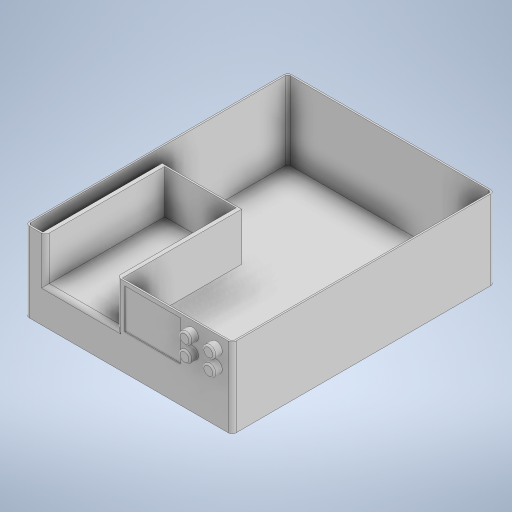
# Autodesk Inventor part: case_botten
Saved by Autodesk Inventor 2023 (Build 270158000, 158)
## iProperties
Created: 2022-12-13
Part Number: case_botten
Material: Generic
Document SubType Name: Modeling
Designer: abdul
Density: 1 g/cm^3
Appearance: Default
Author: abdul
Autodesk Inventor part; units mm, degrees
ref_plane "YZ Plane" through (0, 0, 0) normal (1, 0, 0) x (0, 1, 0)
ref_plane "XZ Plane" through (0, 0, 0) normal (0, 1, 0) x (-1, 0, 0)
ref_plane "XY Plane" through (0, 0, 0) normal (0, 0, 1) x (1, 0, 0)
sketch "Sketch1" plane through (0, 0, 0) normal (0, 1, 0) x (-1, 0, 0)
  line L0 (130, 165) -> (-130, 165)
  line L1 (-130, 165) -> (-130, -165)
  line L2 (-130, -165) -> (130, -165)
  line L3 (130, -165) -> (130, 165)
  point P0 (0, 0)
  point P1 (0, -165)
  point P2 (130, 0)
  dimension "d0" = 260
  dimension "d1" = 330
  constraints: 8 end point, 2 midpoint, 2 parallel, 1 horizontal, 1 horizontal alignment, 1 perpendicular, 1 vertical alignment
  measures "d0" distance of L2.end L1.end
  measures "d1" distance of L1.end L0.end
extrude "Extrusion1" add sketch "Sketch1" along normal blind 100
fillet "Fillet1" radius 5 4 edges at (130, 50, 165) (130, 50, -165) (-130, 50, -165) (-130, 50, 165)
shell "Shell1" thickness 2 removed faces 1 at (43.3333, 100, 53.3333)
sketch "Sketch3" plane through (128, 96, 163) normal (0, 0, -1) x (-1, 0, 0)
  line L0 (251.5, 4) -> (4.5, 4) projected
  line L1 (138, 4) -> (238, 4)
  line L2 (238, 4) -> (238, -56)
  line L3 (238, -56) -> (138, -56)
  line L4 (138, -56) -> (138, 4)
  line L5 (253, -96) -> (253, 4) projected
  point P0 (128, -96)
  point P1 (253, 2)
  dimension "d13" = 100
  dimension "d14" = 60
  dimension "d15" = 15
  constraints: 8 end point, 2 parallel, 1 horizontal, 1 perpendicular, 1 point on line
  measures "d13" distance of L2.end L3.end
  measures "d14" distance of L1.end L2.end
  measures "d15" distance between parallel lines of L2 L5
extrude "Extrusion3" add sketch "Sketch3" along normal blind 150
sketch "Sketch4" plane through (-125, 0, 165) normal (0, 0, 1) x (1, 0, 0)
  line L0 (0, 0) -> (0, 100) projected
  line L1 (0, 0) -> (250, 0) projected
  line L2 (250, 100) -> (250, 0) projected
  line L3 (15, 100) -> (115, 100) projected
  line L4 (15, 40) -> (15, 100) projected
  line L5 (15, 100) -> (115, 100) projected
  line L6 (115, 100) -> (115, 40) projected
  line L7 (115, 40) -> (15, 40) projected
  line L8 (20, 45) -> (110, 45)
  line L9 (110, 45) -> (110, 109.7523)
  line L10 (110, 109.7523) -> (20, 109.7523)
  line L11 (20, 109.7523) -> (20, 45)
  line L12 (0, 100) -> (250, 100) projected
  line L13 (0, 100) -> (-3, 100) projected
  line L14 (-3, 100) -> (0, 100) projected
  line L15 (0, 100) -> (250, 100) projected
  line L16 (250, 100) -> (253, 100) projected
  line L17 (253, 100) -> (250, 100) projected
  line L18 (250, 100) -> (115, 100) projected
  line L19 (15, 100) -> (0, 100) projected
  point P0 (125, 0)
  dimension "d18" = 5
  dimension "d19" = 5
  dimension "d20" = 5
  constraints: 8 end point, 2 parallel, 1 horizontal, 1 perpendicular
  measures "d18" distance between parallel lines of L8 L7
  measures "d19" distance between parallel lines of L4 L11
  measures "d20" distance between parallel lines of L6 L9
extrude "Extrusion4" cut sketch "Sketch4" against normal blind 150 contours L11 L10 L9 L3 | L3 L9 L8 L11
fillet "Fillet3" radius 5 3 edges at (-60, 45, 165) (-105, 72.5, 165) (-15, 72.5, 165)
sketch "Sketch5" plane through (-125, 0, 165) normal (0, 0, 1) x (1, 0, 0)
  circle A0 centre (235, 85) radius 7.5
  line L0 (115, 100) -> (250, 100) projected
  line L1 (250, 100) -> (250, 0) projected
  circle A1 centre (205, 85) radius 7.5
  circle A2 centre (235, 65) radius 7.5
  circle A3 centre (205, 65) radius 7.5
  point P0 (125, 0)
  dimension "d24" = 15
  dimension "d25" = 15
  dimension "d26" = 15
  dimension "d29" = 30
  dimension "d32" = 20
  constraints: 4 centre point, 1 horizontal, 1 vertical, 6 other
  measures "d24" diameter of A0
  measures "d25" distance from line of L0 A0.centre
  measures "d26" distance from line of L1 A0.centre
  measures "d29" distance of A0.centre A1.centre
  measures "d32" distance of A0.centre A2.centre
extrude "Extrusion5" add sketch "Sketch5" along normal blind 10
fillet "Fillet4" radius 2 4 edges at (102.5, 85, 175) (102.5, 65, 175) (72.5, 65, 175) (72.5, 85, 175)
sketch "Sketch6" plane through (-125, 0, 165) normal (0, 0, 1) x (1, 0, 0)
  line L0 (120, 95) -> (190, 95)
  line L1 (190, 95) -> (190, 45)
  line L2 (190, 45) -> (120, 45)
  line L3 (120, 45) -> (120, 95)
  line L4 (115, 100) -> (250, 100) projected
  line L5 (115, 40) -> (115, 100) projected
  point P0 (125, 0)
  dimension "d38" = 5
  dimension "d39" = 5
  dimension "d40" = 70
  dimension "d41" = 50
  constraints: 8 end point, 2 parallel, 1 horizontal, 1 perpendicular
  measures "d38" distance between parallel lines of L4 L0
  measures "d39" distance between parallel lines of L5 L3
  measures "d40" distance of L1.end L2.end
  measures "d41" distance of L0.end L1.end
extrude "Extrusion6" cut sketch "Sketch6" against normal blind 1
body "Solid1"
